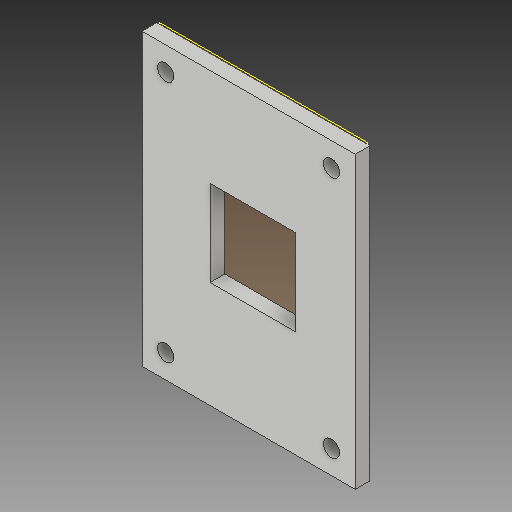
# Autodesk Inventor part: Pieza5
Saved by Autodesk Inventor 2017 (Build 210142000, 142)
## iProperties
Part Number: Pieza5
Material: Genérico
Document SubType Name: Modeling
Designer: user
Density: 1 g/cm^3
Appearance: Valor por defecto
Author: user
Autodesk Inventor part; units mm, degrees
ref_plane "YZ Plane" through (0, 0, 0) normal (1, 0, 0) x (0, 1, 0)
ref_plane "XZ Plane" through (0, 0, 0) normal (0, 1, 0) x (-1, 0, 0)
ref_plane "XY Plane" through (0, 0, 0) normal (0, 0, 1) x (1, 0, 0)
ref_plane "Plano de trabajo1" through (0, 0, 0) normal (0, 0, 1) x (1, 0, 0)
sketch "Boceto1" plane through (0, 0, 0) normal (0, 0, 1) x (1, 0, 0)
  line L0 (-11.9558, -9.942) -> (-11.9558, 34.058) projected
  line L1 (-11.9558, 34.058) -> (15.0442, 34.058) projected
  line L2 (15.0442, 34.058) -> (15.0442, 19.058) projected
  line L3 (15.0442, 19.058) -> (17.0442, 19.058) projected
  line L4 (17.0442, 19.058) -> (17.0442, -9.942) projected
  line L5 (17.0442, -9.942) -> (-11.9558, -9.942) projected
  line L6 (5.0442, -14.942) -> (5.0442, -45.942) projected
  line L7 (5.0442, -45.942) -> (37.0442, -45.942) projected
  line L8 (37.0442, -45.942) -> (37.0442, 52.058) projected
  line L9 (37.0442, 52.058) -> (-34.9558, 52.058) projected
  line L10 (-34.9558, 52.058) -> (-34.9558, -45.942) projected
  line L11 (-34.9558, -45.942) -> (-16.9558, -45.942) projected
  line L12 (-16.9558, -45.942) -> (-16.9558, -14.942) projected
  line L13 (-16.9558, -14.942) -> (5.0442, -14.942) projected
  line L14 (-20.9558, -31.942) -> (-20.9558, 38.058) projected
  line L15 (-20.9558, 38.058) -> (23.0442, 38.058) projected
  line L16 (23.0442, 38.058) -> (23.0442, -31.942) projected
  line L17 (23.0442, -31.942) -> (-20.9558, -31.942) projected
  line L18 (-34.9558, -45.942) -> (37.0442, -45.942) projected
  line L19 (37.0442, -45.942) -> (37.0442, 52.058) projected
  line L20 (37.0442, 52.058) -> (-34.9558, 52.058) projected
  line L21 (-34.9558, 52.058) -> (-34.9558, -45.942) projected
  line L22 (-34.9558, -45.942) -> (37.0442, -45.942)
  line L23 (37.0442, -45.942) -> (37.0442, 52.058)
  line L24 (37.0442, 52.058) -> (-34.9558, 52.058)
  line L25 (-34.9558, 52.058) -> (-34.9558, -45.942)
  line L26 (-11.9558, -9.942) -> (17.0442, -9.942)
  line L27 (17.0442, -9.942) -> (17.0442, 19.058)
  line L28 (17.0442, 19.058) -> (-11.9558, 19.058)
  line L29 (-11.9558, 19.058) -> (-11.9558, -9.942)
  circle A0 centre (29.0442, -37.942) radius 2.75 projected
  circle A1 centre (-26.9558, 44.058) radius 2.75 projected
  circle A2 centre (29.0442, 44.058) radius 2.75 projected
  circle A3 centre (-26.9558, -37.942) radius 2.75 projected
  circle A4 centre (29.0442, -37.942) radius 2.75 projected
  circle A5 centre (-26.9558, 44.058) radius 2.75 projected
  circle A6 centre (29.0442, 44.058) radius 2.75 projected
  circle A7 centre (-26.9558, -37.942) radius 2.75 projected
  point P0 (0, 0)
  constraints: 16 end point, 4 parallel, 2 horizontal, 2 perpendicular
extrude "Extrusión1" add sketch "Boceto1" along normal blind 5 contours L0 L1 L2 L28 | L13 L12 L17 L14 L15 L16 L6 | L6 L17 L12 L13 | L17 L16 L15 L14 L12 L11 L10 L9 L8 L7 L6 | L6 L18 L12 L17 | A0 | A1 | A2 | A3
sketch "Boceto2" plane through (0, 0, 5) normal (0, 0, 1) x (1, 0, 0)
  point P0 (-26.9558, 44.058)
  point P1 (29.0442, 44.058)
  point P2 (29.0442, -37.942)
  point P3 (-26.9558, -37.942)
hole "Agujero1" at (-26.9558, 44.058, 5) at (29.0442, 44.058, 5) at (29.0442, -37.942, 5) at (-26.9558, -37.942, 5) direction (0, 0, -1) diameter 5.5 depth 5
